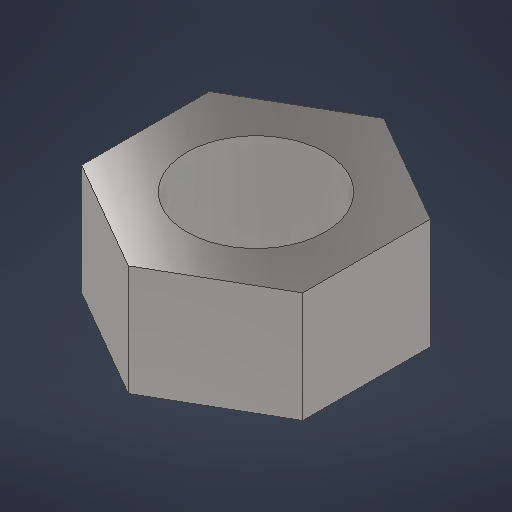
# Autodesk Inventor part: 01-03-01 Kugellager
Saved by Autodesk Inventor 2026.2 (Build 302298000, 298)
## iProperties
Created: 2025-12-11
Part Number: 01-03-01 Kugellager
Material: Stahl, Guss
Document SubType Name: Modeling
Designer: Schally
Density: 7.85 g/cm^3
Appearance: Halbpoliert
Author: Schally
Autodesk Inventor part; units mm, degrees
ref_plane "YZ Plane" through (0, 0, 0) normal (1, 0, 0) x (0, 1, 0)
ref_plane "XZ Plane" through (0, 0, 0) normal (0, 1, 0) x (-1, 0, 0)
ref_plane "XY Plane" through (0, 0, 0) normal (0, 0, 1) x (1, 0, 0)
sketch "Skizze3" plane through (0, 0, 0) normal (0, 1, 0) x (-1, 0, 0)
  circle A0 centre (0, 0) radius 2.5
  line L0 (4, 0) -> (4, 9.599)
  line L1 (4, 9.599) -> (4, -8.7779)
  line L2 (-4, 0) -> (-4, 9.2876)
  line L3 (-4, 9.2876) -> (-4, -8.3814)
  line L4 (-6.313, 8.2636) -> (9.6019, -0.9248)
  line L5 (-10.313, -1.3354) -> (5.6019, 7.853)
  line L6 (-4, -9.599) -> (-4, 8.7779)
  line L7 (6.313, -8.2636) -> (-9.6019, 0.9248)
  line L8 (10.313, 1.3354) -> (-5.6019, -7.853)
  point P0 (0, -4.6188)
  point P1 (4, -2.3094)
  point P2 (4, 2.3094)
  point P3 (0, 4.6188)
  point P4 (-4, 2.3094)
  point P5 (-4, -2.3094)
  dimension "d34" = 5
  dimension "d38" = 360
  constraints: 18 end point, 2 point on line, 2 vertical, 1 centre point, 1 coincident, 19 other
  measures "d34" diameter of A0
extrude "Extrusion1" add sketch "Skizze3" along normal blind 4 contours L1 L8 L7 L3 L2 L5 L4 L0
